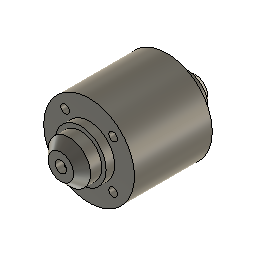
Mecanum Wheel Assembly (Autodesk Fusion 360 archive; units mm, degrees)
design "Internal connector"
Autodesk Fusion 360 part; units mm, degrees
sketch "Sketch1" plane through (0, 0, 0) normal (0, 1, 0) x (1, 0, 0)
  circle A0 centre (0, 0) radius 16
  dimension "d1" = 32
  constraint coincident A0.centre origin
  measures "d1" diameter of A0
extrude "Extrude1" add sketch "Sketch1" along normal blind 27.5 makes body 1
sketch "Sketch2" plane through (0, 0, 0) normal (0, -1, 0) x (1, 0, 0)
  circle A0 centre (0, 0) radius 16
  circle A1 centre (0, 0) radius 9
  dimension "d4" = 18
  constraint coincident A0.centre A1.centre
  measures "d4" diameter of A1
extrude "Extrude2" add sketch "Sketch2" along normal blind 3 contours A1 bodies 1
extrude "Extrude3" add 1 faces at (-3.8718, -3, 0.199) along direction (0, 1, 0) blind 3 from surface at 30.5 on bodies 1 bodies 1
sketch "Sketch3" plane through (0, 30.5, 0) normal (0, 1, 0) x (-1, 0, 0)
  circle A0 centre (0, 0) radius 9
  circle A1 centre (0, 0) radius 7.5
  dimension "d10" = 15
  constraint coincident A0.centre A1.centre
  measures "d10" diameter of A1
extrude "Extrude4" add sketch "Sketch3" along normal blind 7 contours A1 bodies 1
sketch "Sketch4" plane through (0, 37.5, 0) normal (0, 1, 0) x (-1, 0, 0)
  circle A0 centre (0, 0) radius 7.5
  circle A1 centre (0, 0) radius 1.5
  dimension "d13" = 3
  constraint coincident A0.centre A1.centre
  measures "d13" diameter of A1
extrude "Extrude5" cut sketch "Sketch4" against normal blind 5 contours A1 bodies 1
chamfer "Chamfer1" distance 3 angle 45 1 edges at (6.9925, 37.5, -2.7121) on bodies 1
ref_plane "WorkPlane1" through (0, 13.75, 0) normal (0, -1, 0) x (-1, 0, 0)
split "Split1" by plane through (0, 13.75, 0) normal (0, -1, 0) bodies 1 makes body 2 at (15.9205, 9.1667, -1.5931)
delete_body "RemoveBody1" bodies 2
mirror "Mirror1" about plane through (0, 13.75, 0) normal (0, -1, 0) of bodies 1 merged
sketch "Sketch5" plane through (0, 0, 0) normal (0, -1, 0) x (1, 0, 0)
  circle A0 centre (0, 0) radius 9
  circle A1 centre (0, 0) radius 16
  circle A2 centre (0, 0) radius 12 construction
  line L0 (0, 0) -> (0, 20) construction
  line L1 (0, 0) -> (-16.9706, 16.9706) construction
  circle A3 centre (-8.4853, 8.4853) radius 1.5
  circle A4 centre (-8.4853, -8.4853) radius 1.5
  circle A5 centre (8.4853, -8.4853) radius 1.5
  circle A6 centre (8.4853, 8.4853) radius 1.5
  dimension "d20" = 24
  dimension "d21" = 45
  dimension "d22" = 3
  dimension "d24" = 360
  constraint coincident A0.centre A1.centre
  constraint vertical L0
  constraint midpoint L1 A3.centre
  constraint coincident A2 A3.centre
  measures "d20" diameter of A2
  measures "d21" angle of L0 L1
  measures "d22" diameter of A3
extrude "Extrude6" cut sketch "Sketch5" against normal blind 35 contours A3 | A4 | A5 | A6 bodies 1
sketch "Sketch6" plane through (0, -10, 0) normal (0, -1, 0) x (1, 0, 0)
  circle A0 centre (0, 0) radius 1.5
  circle A1 centre (0, 0) radius 4.5
  circle A2 centre (0, 0) radius 2
  line L0 (0, 2) -> (0, -1.5) construction
  line L1 (-1.3229, -1.5) -> (1.3229, -1.5)
  dimension "d27" = 4
  dimension "d28" = 3.5
  constraint coincident A0.centre A1.centre
  constraint coincident A2 L0.start
  constraint vertical L0
  constraint perpendicular L0 L1
  constraint coincident A2 L1.start
  constraint coincident L0.end L1
  constraint coincident A2 L1.end
  constraint midpoint L0.end L1
  measures "d27" diameter of A2
  measures "d28" distance of L0.start L0.end
extrude "Extrude7" cut sketch "Sketch6" against normal blind 50 contours A0 | A2 L1 picked at (-1.2865, -1.3001) bodies 1
extrude "Extrude8" cut sketch "Sketch6" against normal blind 2.5 contours A2 L1 picked at (0.096, -1.8264) bodies 1
mirror "Mirror2" about plane through (0, 13.75, 0) normal (0, -1, 0) of "Extrude8"
equation "d17 = ( -27.50 / 2 ) * 1 mm"

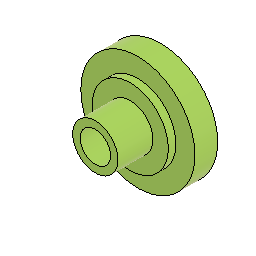
design "Roller joint"
Autodesk Fusion 360 part; units mm, degrees
sketch "Sketch1" plane through (0, 0, 0) normal (0, 1, 0) x (1, 0, 0)
  circle A0 centre (0, 0) radius 3.75
  dimension "d1" = 7.5
  constraint coincident A0.centre origin
  measures "d1" diameter of A0
extrude "Extrude1" add sketch "Sketch1" along normal blind 1.5
sketch "Sketch2" plane through (0, 0, 0) normal (0, -1, 0) x (1, 0, 0)
  circle A0 centre (0, 0) radius 3.75
  circle A1 centre (0, 0) radius 2.5
  dimension "d4" = 5
  constraint coincident A0.centre A1.centre
  measures "d4" diameter of A1
extrude "Extrude2" add sketch "Sketch2" along normal blind 0.5 contours A1
sketch "Sketch3" plane through (0, -0.5, 0) normal (0, -1, 0) x (1, 0, 0)
  circle A0 centre (0, 0) radius 2.5
  circle A1 centre (0, 0) radius 1.4875
  dimension "d7" = 2.975
  constraint coincident A0.centre A1.centre
  measures "d7" diameter of A1
extrude "Extrude3" add sketch "Sketch3" along normal blind 0.8 contours A1
sketch "Sketch4" plane through (0, -1.3, 0) normal (0, -1, 0) x (1, 0, 0)
  circle A0 centre (0, 0) radius 1.4875
  circle A1 centre (0, 0) radius 1
  dimension "d10" = 2
  constraint coincident A0.centre A1.centre
  measures "d10" diameter of A1
extrude "Extrude4" cut sketch "Sketch4" against normal blind 6.5 contours A1
extrude "Extrude5" add 1 faces at (1.3157, -1.3, -0.1236) along direction (0, -1, 0) blind 1.5

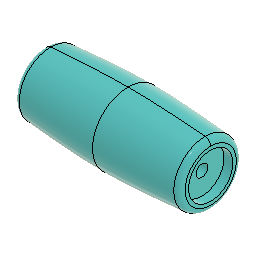
design "Roller"
Autodesk Fusion 360 part; units mm, degrees
sketch "Sketch1" plane through (0, 0, 0) normal (0, 1, 0) x (1, 0, 0)
  line L0 (0, -5) -> (0, 5) construction
  line L1 (-5, 0) -> (5, 0) construction
  line L2 (0, -1) -> (12.5, -1)
  line L3 (12.5, -1) -> (12.5, -3.75)
  line L4 (12.5, -3.75) -> (14, -3.75)
  line L5 (14, -3.75) -> (14, -5.25)
  spline S0 degree 5 poles (14, -5.25) (13.4403, -5.2966) (12.3208, -5.388) (10.6416, -5.5192) (8.4023, -5.6817) (5.6027, -5.8541) (3.3623, -5.9519) (1.6814, -5.9912) (0.5605, -6) (0, -6) knots 0 0 0 0 0 0 0.2 0.4 0.6 0.8 1 1 1 1 1 1
  line L6 (1.428, -6) -> (-1.428, -6)
  spline S1 degree 5 poles (-14, -5.25) (-13.4403, -5.2966) (-12.3208, -5.388) (-10.6416, -5.5192) (-8.4023, -5.6817) (-5.6027, -5.8541) (-3.3623, -5.9519) (-1.6814, -5.9912) (-0.5605, -6) (0, -6) knots 0 0 0 0 0 0 0.2 0.4 0.6 0.8 1 1 1 1 1 1
  line L7 (15.4266, -5.1311) -> (12.5734, -5.3689)
  line L8 (-15.4266, -5.1311) -> (-12.5734, -5.3689)
  line L9 (-1.428, -6) -> (1.428, -6)
  line L10 (0, -1) -> (-12.5, -1)
  line L11 (-12.5, -1) -> (-12.5, -3.75)
  line L12 (-12.5, -3.75) -> (-14, -3.75)
  line L13 (-14, -3.75) -> (-14, -5.25)
  dimension "d1" = 1.5
  dimension "d2" = 1.5
  dimension "d3" = 14
  dimension "d5" = 6
  dimension "d6" = 3.75
  constraint vertical L0
  constraint horizontal L1
  constraint coincident L0 L2.start
  constraint perpendicular L0 L2
  constraint perpendicular L2 L3
  constraint perpendicular L0 L4
  constraint perpendicular L4 L5
  constraint coincident origin L1
  constraint midpoint L0 L1
  constraint coincident L0 S0.end
  constraint midpoint S0.end L6
  constraint horizontal L6
  constraint coincident origin L0
  constraint midpoint L5.end L7
  constraint symmetric L0 L2.start L10.start
  constraint symmetric L0 L2.end L10.end
  constraint symmetric L0 L3.end L11.end
  constraint symmetric L0 L4.end L12.end
  constraint symmetric L0 L5.end S1.start
  constraint symmetric L0 S0.end S1.end
  constraint symmetric L0 L6.start L6.end
  constraint symmetric L0 L6.end L6.start
  constraint symmetric L0 L7.start L8.start
  constraint symmetric L0 L7.end L8.end
  measures "d1" distance of L3.end L4.end
  measures "d2" distance of L4.end L5.end
  measures "d3" distance of L0 L5.end
  measures "d5" distance of origin S0.end
  measures "d6" distance of L1 L3.end
revolve "Revolve1" add sketch "Sketch1" angle 360 about axis through (-5, 0, 0) along (1, 0, 0)
fillet "Fillet1" radius 1 2 edges at (14, -1.8985, -4.8947) (-14, -1.8985, -4.8947)
named bodies: "Roller"

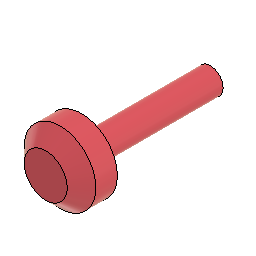
design "miniwheel connector pin"
Autodesk Fusion 360 part; units mm, degrees
sketch "Sketch1" plane through (0, 0, 0) normal (0, 1, 0) x (1, 0, 0)
  circle A0 centre (0, 0) radius 2.5
  dimension "d1" = 5
  constraint coincident A0.centre origin
  measures "d1" diameter of A0
extrude "Extrude1" add sketch "Sketch1" along normal blind 2.5
chamfer "Chamfer1" distance 1 angle 45 1 edges at (-2.3308, 0, 0.904)
sketch "Sketch2" plane through (0, 2.5, 0) normal (0, 1, 0) x (-1, 0, 0)
  circle A0 centre (0, 0) radius 2.5
  circle A1 centre (0, 0) radius 0.9
  dimension "d5" = 1.8
  constraint coincident A0.centre A1.centre
  measures "d5" diameter of A1
extrude "Extrude2" add sketch "Sketch2" along normal blind 9 contours A1
named bodies: "Miniwheel Connector pin"
